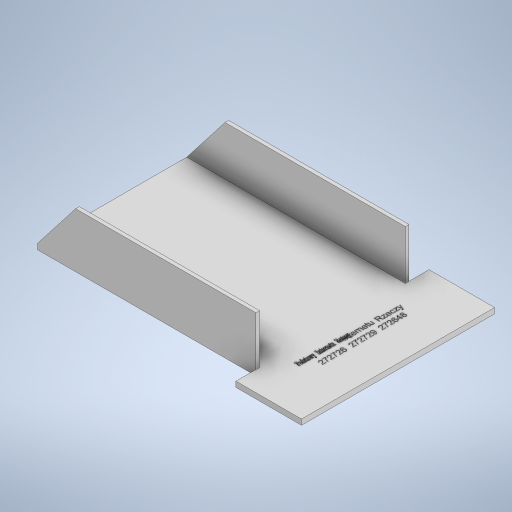
# Autodesk Inventor part: Część1
Saved by Autodesk Inventor 2024 (Build 280153020, 153B)
## iProperties
Created: 2025-01-23
Part Number: Część1
Material: Ogólny
Document SubType Name: Modeling
Designer: jakub
Density: 1 g/cm^3
Appearance: Domyślna
Author: jakub
Autodesk Inventor part; units mm, degrees
(part 1 of 2)
ref_plane "YZ Plane" through (0, 0, 0) normal (1, 0, 0) x (0, 1, 0)
ref_plane "XZ Plane" through (0, 0, 0) normal (0, 1, 0) x (-1, 0, 0)
ref_plane "XY Plane" through (0, 0, 0) normal (0, 0, 1) x (1, 0, 0)
sketch "Szkic1" plane through (0, 0, 0) normal (0, 1, 0) x (-1, 0, 0)
  line L0 (-24, 40) -> (60, 40)
  line L1 (60, -40) -> (-24, -40)
  line L2 (-60, -40) -> (-60, 40)
  line L3 (-60, 40) -> (60, -40) construction
  line L4 (60, 40) -> (-60, -40) construction
  line L5 (-24, -40) -> (-24, -53)
  line L6 (-24, -53) -> (-60, -53)
  line L7 (-60, -53) -> (-60, -40)
  line L8 (-24, 40) -> (-24, 53)
  line L9 (-24, 53) -> (-60, 53)
  line L10 (-60, 53) -> (-60, 40)
  line L11 (60, -40) -> (96, -40)
  line L12 (96, -40) -> (96, 40)
  line L13 (96, 40) -> (60, 40)
  point P0 (0, 0)
  dimension "d0" = 120
  dimension "d1" = 80
  dimension "d6" = 106
  dimension "d7" = 84
  dimension "d8" = 84
  dimension "d9" = 13
  dimension "d10" = 13
  dimension "d11" = 40
  dimension "d12" = 53
  dimension "d16" = 36
  dimension "d17" = 80
  dimension "d18" = 156
  constraints: 28 end point, 4 parallel, 2 horizontal, 2 midpoint, 1 perpendicular
  measures "d0" distance of L1.start L2.start
  measures "d1" distance of L0.end L1.start
  measures "d6" distance between parallel lines of L6 L9
  measures "d7" distance of L0.start L0.end
  measures "d8" distance of L1.start L1.end
  measures "d9" distance of L0.start L8.end
  measures "d10" distance of L1.end L5.end
  measures "d11" distance from line of point (0, 0) L1
  measures "d12" distance from line of point (0, 0) L9
  measures "d16" distance of L13.end L12.end
  measures "d17" distance of L11.end L12.end
  measures "d18" distance between parallel lines of L2 L12
extrude "Wyciągnięcie proste1" add sketch "Szkic1" along normal blind 3
sketch "Szkic2" plane through (0, 0, 0) normal (0, -1, 0) x (1, 0, 0)
  line L0 (24, -40) -> (-96, -40)
  line L1 (-96, -40) -> (-96, -42)
  line L2 (-96, -42) -> (24, -42)
  line L3 (24, -42) -> (24, -40)
  line L4 (24, 40) -> (-96, 40)
  line L5 (-96, 40) -> (-96, 42)
  line L6 (-96, 42) -> (24, 42)
  line L7 (24, 42) -> (24, 40)
  point P0 (0, 0)
  dimension "d19" = 2
  dimension "d20" = 120
  dimension "d21" = 2
  constraints: 16 end point, 4 parallel, 2 horizontal, 2 perpendicular, 1 point on line
  measures "d19" distance of L1.end L0.end
  measures "d20" distance of L5.end L6.end
  measures "d21" distance of L4.end L5.end
extrude "Wyciągnięcie proste2" add sketch "Szkic2" against normal blind 30
sketch "Szkic4" plane through (0, 3, 0) normal (0, 1, 0) x (1, 0, 0)
  line L0 (34.7111, -3.5872) -> (31.6611, -3.5872)
  line L1 (31.6611, -3.5872) -> (31.6611, -3.1828)
  line L2 (31.6611, -3.1828) -> (34.7111, -3.1828)
  line L3 (34.7111, -3.1828) -> (34.7111, -3.5872)
  line L4 (34.7111, -2.5202) -> (32.5003, -2.5202)
  line L5 (32.5003, -2.5202) -> (32.5003, -2.1831)
  line L6 (32.5003, -2.1831) -> (32.8141, -2.1831)
  spline S0 degree 2 poles (32.8141, -2.1831) (32.4515, -1.939) (32.4515, -1.4811) knots 0 0 0 1 1 1
  spline S1 degree 2 poles (32.4515, -1.4811) (32.4515, -1.2811) (32.5956, -0.9464) (32.8281, -0.779) (32.9885, -0.7465) knots 0 0 0 1 2 3 3 3
  spline S2 degree 2 poles (32.9885, -0.7465) (33.0931, -0.7255) (33.3534, -0.7255) knots 0 0 0 1 1 1
  line L7 (33.3534, -0.7255) -> (34.7111, -0.7255)
  line L8 (34.7111, -0.7255) -> (34.7111, -1.0998)
  line L9 (34.7111, -1.0998) -> (33.3674, -1.0998)
  spline S3 degree 2 poles (33.3674, -1.0998) (33.1396, -1.0998) (32.9117, -1.1882) (32.7769, -1.409) (32.7769, -1.5601) knots 0 0 0 1 2 3 3 3
  spline S4 degree 2 poles (32.7769, -1.5601) (32.7769, -1.7996) (33.0814, -2.1459) (33.5045, -2.1459) knots 0 0 0 1 2 2 2
  line L10 (33.5045, -2.1459) -> (34.7111, -2.1459)
  line L11 (34.7111, -2.1459) -> (34.7111, -2.5202)
  line L12 (34.3763, 0.6646) -> (34.7087, 0.7181)
  spline S5 degree 2 poles (34.7087, 0.7181) (34.7413, 0.56) (34.7413, 0.4345) knots 0 0 0 1 1 1
  spline S6 degree 2 poles (34.7413, 0.4345) (34.7413, 0.2322) (34.6111, 0.0067) (34.4019, -0.0839) (34.0648, -0.0839) knots 0 0 0 1 2 3 3 3
  line L13 (34.0648, -0.0839) -> (32.7909, -0.0839)
  line L14 (32.7909, -0.0839) -> (32.7909, -0.3606)
  line L15 (32.7909, -0.3606) -> (32.5003, -0.3606)
  line L16 (32.5003, -0.3606) -> (32.5003, -0.0839)
  line L17 (32.5003, -0.0839) -> (31.954, -0.0839)
  line L18 (31.954, -0.0839) -> (31.7285, 0.2903)
  line L19 (31.7285, 0.2903) -> (32.5003, 0.2903)
  line L20 (32.5003, 0.2903) -> (32.5003, 0.6646)
  line L21 (32.5003, 0.6646) -> (32.7909, 0.6646)
  line L22 (32.7909, 0.6646) -> (32.7909, 0.2903)
  line L23 (32.7909, 0.2903) -> (34.0857, 0.2903)
  spline S7 degree 2 poles (34.0857, 0.2903) (34.2461, 0.2903) (34.3391, 0.3299) (34.3926, 0.4182) (34.3926, 0.5019) knots 0 0 0 1 2 3 3 3
  spline S8 degree 2 poles (34.3926, 0.5019) (34.3926, 0.5623) (34.3763, 0.6646) knots 0 0 0 1 1 1
  line L24 (33.9974, 2.543) -> (34.0462, 2.9312)
  spline S9 degree 2 poles (34.0462, 2.9312) (34.3856, 2.8382) (34.7599, 2.3431) (34.7599, 1.9595) knots 0 0 0 1 2 2 2
  spline S10 degree 2 poles (34.7599, 1.9595) (34.7599, 1.4736) (34.1624, 0.9064) (33.6254, 0.9064) knots 0 0 0 1 2 2 2
  spline S11 degree 2 poles (33.6254, 0.9064) (33.0675, 0.9064) (32.4515, 1.4806) (32.4515, 1.9386) knots 0 0 0 1 2 2 2
  spline S12 degree 2 poles (32.4515, 1.9386) (32.4515, 2.3802) (33.0559, 2.9428) (33.6022, 2.9428) knots 0 0 0 1 2 2 2
  spline S13 degree 2 poles (33.6022, 2.9428) (33.6347, 2.9428) (33.7021, 2.9405) knots 0 0 0 1 1 1
  line L25 (33.7021, 2.9405) -> (33.7021, 1.2923)
  spline S14 degree 2 poles (33.7021, 1.2923) (34.0671, 1.3132) (34.453, 1.6828) (34.453, 1.9595) knots 0 0 0 1 2 2 2
  spline S15 degree 2 poles (34.453, 1.9595) (34.453, 2.1664) (34.2345, 2.457) (33.9974, 2.543) knots 0 0 0 1 2 2 2
  line L26 (33.3953, 1.3132) -> (33.3953, 2.5476)
  spline S16 degree 2 poles (33.3953, 2.5476) (33.1163, 2.5221) (32.9745, 2.4058) knots 0 0 0 1 1 1
  spline S17 degree 2 poles (32.9745, 2.4058) (32.7583, 2.2268) (32.7583, 1.9409) knots 0 0 0 1 1 1
  spline S18 degree 2 poles (32.7583, 1.9409) (32.7583, 1.6828) (33.1047, 1.3318) (33.3953, 1.3132) knots 0 0 0 1 2 2 2
  line L27 (34.7111, 3.3961) -> (32.5003, 3.3961)
  line L28 (32.5003, 3.3961) -> (32.5003, 3.7332)
  line L29 (32.5003, 3.7332) -> (32.835, 3.7332)
  spline S19 degree 2 poles (32.835, 3.7332) (32.6002, 3.8611) (32.4515, 4.0796) (32.4515, 4.2121) knots 0 0 0 1 2 2 2
  spline S20 degree 2 poles (32.4515, 4.2121) (32.4515, 4.4004) (32.57, 4.5957) knots 0 0 0 1 1 1
  line L30 (32.57, 4.5957) -> (32.9187, 4.4655)
  spline S21 degree 2 poles (32.9187, 4.4655) (32.8374, 4.3283) (32.8374, 4.1912) knots 0 0 0 1 1 1
  spline S22 degree 2 poles (32.8374, 4.1912) (32.8374, 4.068) (32.9861, 3.875) (33.1163, 3.8332) knots 0 0 0 1 2 2 2
  spline S23 degree 2 poles (33.1163, 3.8332) (33.3162, 3.7704) (33.5534, 3.7704) knots 0 0 0 1 1 1
  line L31 (33.5534, 3.7704) -> (34.7111, 3.7704)
  line L32 (34.7111, 3.7704) -> (34.7111, 3.3961)
  line L33 (34.7111, 4.8189) -> (32.5003, 4.8189)
  line L34 (32.5003, 4.8189) -> (32.5003, 5.1559)
  line L35 (32.5003, 5.1559) -> (32.8141, 5.1559)
  spline S24 degree 2 poles (32.8141, 5.1559) (32.4515, 5.4) (32.4515, 5.858) knots 0 0 0 1 1 1
  spline S25 degree 2 poles (32.4515, 5.858) (32.4515, 6.0579) (32.5956, 6.3927) (32.8281, 6.56) (32.9885, 6.5926) knots 0 0 0 1 2 3 3 3
  spline S26 degree 2 poles (32.9885, 6.5926) (33.0931, 6.6135) (33.3534, 6.6135) knots 0 0 0 1 1 1
  line L36 (33.3534, 6.6135) -> (34.7111, 6.6135)
  line L37 (34.7111, 6.6135) -> (34.7111, 6.2392)
  line L38 (34.7111, 6.2392) -> (33.3674, 6.2392)
  spline S27 degree 2 poles (33.3674, 6.2392) (33.1396, 6.2392) (32.9117, 6.1509) (32.7769, 5.9301) (32.7769, 5.7789) knots 0 0 0 1 2 3 3 3
  spline S28 degree 2 poles (32.7769, 5.7789) (32.7769, 5.5395) (33.0814, 5.1931) (33.5045, 5.1931) knots 0 0 0 1 2 2 2
  line L39 (33.5045, 5.1931) -> (34.7111, 5.1931)
  line L40 (34.7111, 5.1931) -> (34.7111, 4.8189)
  line L41 (33.9974, 8.6988) -> (34.0462, 9.087)
  spline S29 degree 2 poles (34.0462, 9.087) (34.3856, 8.994) (34.7599, 8.4988) (34.7599, 8.1153) knots 0 0 0 1 2 2 2
  spline S30 degree 2 poles (34.7599, 8.1153) (34.7599, 7.6294) (34.1624, 7.0622) (33.6254, 7.0622) knots 0 0 0 1 2 2 2
  spline S31 degree 2 poles (33.6254, 7.0622) (33.0675, 7.0622) (32.4515, 7.6364) (32.4515, 8.0943) knots 0 0 0 1 2 2 2
  spline S32 degree 2 poles (32.4515, 8.0943) (32.4515, 8.536) (33.0559, 9.0986) (33.6022, 9.0986) knots 0 0 0 1 2 2 2
  spline S33 degree 2 poles (33.6022, 9.0986) (33.6347, 9.0986) (33.7021, 9.0963) knots 0 0 0 1 1 1
  line L42 (33.7021, 9.0963) -> (33.7021, 7.4481)
  spline S34 degree 2 poles (33.7021, 7.4481) (34.0671, 7.469) (34.453, 7.8386) (34.453, 8.1153) knots 0 0 0 1 2 2 2
  spline S35 degree 2 poles (34.453, 8.1153) (34.453, 8.3222) (34.2345, 8.6128) (33.9974, 8.6988) knots 0 0 0 1 2 2 2
  line L43 (33.3953, 7.469) -> (33.3953, 8.7034)
  spline S36 degree 2 poles (33.3953, 8.7034) (33.1163, 8.6778) (32.9745, 8.5616) knots 0 0 0 1 1 1
  spline S37 degree 2 poles (32.9745, 8.5616) (32.7583, 8.3826) (32.7583, 8.0967) knots 0 0 0 1 1 1
  spline S38 degree 2 poles (32.7583, 8.0967) (32.7583, 7.8386) (33.1047, 7.4876) (33.3953, 7.469) knots 0 0 0 1 2 2 2
  line L44 (34.3763, 10.3725) -> (34.7087, 10.426)
  spline S39 degree 2 poles (34.7087, 10.426) (34.7413, 10.2679) (34.7413, 10.1424) knots 0 0 0 1 1 1
  spline S40 degree 2 poles (34.7413, 10.1424) (34.7413, 9.9402) (34.6111, 9.7147) (34.4019, 9.624) (34.0648, 9.624) knots 0 0 0 1 2 3 3 3
  line L45 (34.0648, 9.624) -> (32.7909, 9.624)
  line L46 (32.7909, 9.624) -> (32.7909, 9.3474)
  line L47 (32.7909, 9.3474) -> (32.5003, 9.3474)
  line L48 (32.5003, 9.3474) -> (32.5003, 9.624)
  line L49 (32.5003, 9.624) -> (31.954, 9.624)
  line L50 (31.954, 9.624) -> (31.7285, 9.9983)
  line L51 (31.7285, 9.9983) -> (32.5003, 9.9983)
  line L52 (32.5003, 9.9983) -> (32.5003, 10.3725)
  line L53 (32.5003, 10.3725) -> (32.7909, 10.3725)
  line L54 (32.7909, 10.3725) -> (32.7909, 9.9983)
  line L55 (32.7909, 9.9983) -> (34.0857, 9.9983)
  spline S41 degree 2 poles (34.0857, 9.9983) (34.2461, 9.9983) (34.3391, 10.0378) (34.3926, 10.1261) (34.3926, 10.2098) knots 0 0 0 1 2 3 3 3
  spline S42 degree 2 poles (34.3926, 10.2098) (34.3926, 10.2703) (34.3763, 10.3725) knots 0 0 0 1 1 1
  line L56 (34.7111, 12.1858) -> (34.3856, 12.1858)
  spline S43 degree 2 poles (34.3856, 12.1858) (34.7599, 11.9278) (34.7599, 11.4861) knots 0 0 0 1 1 1
  spline S44 degree 2 poles (34.7599, 11.4861) (34.7599, 11.2908) (34.6111, 10.9514) (34.3833, 10.7863) (34.2182, 10.7538) knots 0 0 0 1 2 3 3 3
  spline S45 degree 2 poles (34.2182, 10.7538) (34.109, 10.7306) (33.8695, 10.7306) knots 0 0 0 1 1 1
  line L57 (33.8695, 10.7306) -> (32.5003, 10.7306)
  line L58 (32.5003, 10.7306) -> (32.5003, 11.1048)
  line L59 (32.5003, 11.1048) -> (33.7254, 11.1048)
  spline S46 degree 2 poles (33.7254, 11.1048) (34.0183, 11.1048) (34.1206, 11.1281) knots 0 0 0 1 1 1
  spline S47 degree 2 poles (34.1206, 11.1281) (34.2694, 11.1629) (34.4367, 11.3908) (34.4367, 11.5605) knots 0 0 0 1 2 2 2
  spline S48 degree 2 poles (34.4367, 11.5605) (34.4367, 11.7278) (34.2647, 12.0231) (33.9672, 12.1463) (33.6835, 12.1463) knots 0 0 0 1 2 3 3 3
  line L60 (33.6835, 12.1463) -> (32.5003, 12.1463)
  line L61 (32.5003, 12.1463) -> (32.5003, 12.5206)
  line L62 (32.5003, 12.5206) -> (34.7111, 12.5206)
  line L63 (34.7111, 12.5206) -> (34.7111, 12.1858)
  line L64 (33.4322, -27.6981) -> (34.2484, -27.6981)
  line L65 (34.2484, -27.6981) -> (34.2484, -28.4374)
  line L66 (34.2484, -28.4374) -> (33.4322, -28.4374)
  line L67 (33.4322, -28.4374) -> (33.4322, -28.2904)
  line L68 (33.4322, -28.2904) -> (31.9784, -28.2904)
  line L69 (31.9784, -28.2904) -> (31.9784, -28.4374)
  line L70 (31.9784, -28.4374) -> (31.1984, -28.4374)
  line L71 (31.1984, -28.4374) -> (31.1984, -27.8269)
  spline S49 degree 2 poles (31.1984, -27.8269) (31.1984, -27.4335) (31.5737, -27.1713) (32.1321, -27.1713) knots 0 0 0 1 2 2 2
  spline S50 degree 2 poles (32.1321, -27.1713) (32.6205, -27.1713) (32.9348, -27.4064) (32.9348, -27.7681) knots 0 0 0 1 2 2 2
  line L72 (32.9348, -27.7681) -> (32.9348, -27.8631)
  line L73 (32.9348, -27.8631) -> (33.4322, -27.8631)
  line L74 (33.4322, -27.8631) -> (33.4322, -27.6981)
  line L75 (31.9784, -27.8631) -> (32.6002, -27.8631)
  line L76 (32.6002, -27.8631) -> (32.6002, -27.8314)
  line L77 (32.6002, -27.8314) -> (32.6002, -27.7727)
  spline S51 degree 2 poles (32.6002, -27.7727) (32.6002, -27.5827) (32.304, -27.5827) knots 0 0 0 1 1 1
  spline S52 degree 2 poles (32.304, -27.5827) (31.9784, -27.5827) (31.9784, -27.8021) knots 0 0 0 1 1 1
  line L78 (31.9784, -27.8021) -> (31.9784, -27.8631)
  line L79 (33.5023, -27.0266) -> (32.7675, -27.0266)
  spline S53 degree 2 poles (32.7675, -27.0266) (32.2723, -27.0266) (31.9467, -26.8457) (31.9467, -26.5676) knots 0 0 0 1 2 2 2
  spline S54 degree 2 poles (31.9467, -26.5676) (31.9467, -26.2918) (32.2814, -26.1086) (32.7901, -26.1086) knots 0 0 0 1 2 2 2
  line L80 (32.7901, -26.1086) -> (33.4729, -26.1086)
  line L81 (33.4729, -26.1086) -> (33.6515, -26.1109)
  spline S55 degree 2 poles (33.6515, -26.1109) (34.2755, -26.1109) (34.2755, -26.5744) knots 0 0 0 1 1 1
  spline S56 degree 2 poles (34.2755, -26.5744) (34.2755, -27.0266) (33.5023, -27.0266) knots 0 0 0 1 1 1
  line L82 (33.2129, -26.4274) -> (32.937, -26.4274)
  line L83 (32.937, -26.4274) -> (32.8353, -26.4297)
  line L84 (32.8353, -26.4297) -> (32.7449, -26.4297)
  spline S57 degree 2 poles (32.7449, -26.4297) (32.5572, -26.4297) (32.5572, -26.5653) knots 0 0 0 1 1 1
  spline S58 degree 2 poles (32.5572, -26.5653) (32.5572, -26.7078) (32.9551, -26.7078) knots 0 0 0 1 1 1
  line L85 (32.9551, -26.7078) -> (33.2445, -26.7078)
  spline S59 degree 2 poles (33.2445, -26.7078) (33.6108, -26.7078) (33.6108, -26.5698) knots 0 0 0 1 1 1
  spline S60 degree 2 poles (33.6108, -26.5698) (33.6108, -26.4274) (33.2129, -26.4274) knots 0 0 0 1 1 1
  line L86 (31.1984, -24.9849) -> (33.6063, -24.9849)
  line L87 (33.6063, -24.9849) -> (33.6063, -24.8674)
  line L88 (33.6063, -24.8674) -> (34.2484, -24.8674)
  line L89 (34.2484, -24.8674) -> (34.2484, -25.2495)
  line L90 (34.2484, -25.2495) -> (34.0381, -25.2495)
  spline S61 degree 2 poles (34.0381, -25.2495) (34.0698, -25.2969) (34.1263, -25.3309) knots 0 0 0 1 1 1
  spline S62 degree 2 poles (34.1263, -25.3309) (34.2778, -25.4213) (34.2778, -25.5773) knots 0 0 0 1 1 1
  spline S63 degree 2 poles (34.2778, -25.5773) (34.2778, -25.9051) (33.4819, -25.9051) knots 0 0 0 1 1 1
  line L91 (33.4819, -25.9051) -> (32.8353, -25.9051)
  spline S64 degree 2 poles (32.8353, -25.9051) (31.9467, -25.9051) (31.9467, -25.5818) knots 0 0 0 1 1 1
  spline S65 degree 2 poles (31.9467, -25.5818) (31.9467, -25.4009) (32.1683, -25.3037) knots 0 0 0 1 1 1
  line L92 (32.1683, -25.3037) -> (31.7094, -25.3037)
  line L93 (31.7094, -25.3037) -> (31.7094, -25.4349)
  line L94 (31.7094, -25.4349) -> (31.1984, -25.4349)
  line L95 (31.1984, -25.4349) -> (31.1984, -24.9849)
  spline S66 degree 2 poles (32.5572, -25.4371) (32.5482, -25.5683) (32.8466, -25.5683) knots 0 0 0 1 1 1
  line L96 (32.8466, -25.5683) -> (33.1157, -25.5705)
  line L97 (33.1157, -25.5705) -> (33.3644, -25.5705)
  spline S67 degree 2 poles (33.3644, -25.5705) (33.6741, -25.5705) (33.6673, -25.4371) knots 0 0 0 1 1 1
  spline S68 degree 2 poles (33.6673, -25.4371) (33.6605, -25.315) (33.2084, -25.315) knots 0 0 0 1 1 1
  spline S69 degree 2 poles (33.2084, -25.315) (32.5662, -25.315) (32.5572, -25.4371) knots 0 0 0 1 1 1
  line L98 (31.9784, -23.9223) -> (32.8556, -23.9223)
  line L99 (32.8556, -23.9223) -> (32.8556, -24.1823)
  line L100 (32.8556, -24.1823) -> (32.7946, -24.1823)
  spline S70 degree 2 poles (32.7946, -24.1823) (32.5595, -24.1823) (32.5595, -24.3496) knots 0 0 0 1 1 1
  spline S71 degree 2 poles (32.5595, -24.3496) (32.5595, -24.4807) (32.6906, -24.4807) knots 0 0 0 1 1 1
  spline S72 degree 2 poles (32.6906, -24.4807) (32.8014, -24.4807) (32.8669, -24.3654) knots 0 0 0 1 1 1
  line L101 (32.8669, -24.3654) -> (32.9642, -24.1959)
  spline S73 degree 2 poles (32.9642, -24.1959) (33.1563, -23.868) (33.5656, -23.868) knots 0 0 0 1 1 1
  spline S74 degree 2 poles (33.5656, -23.868) (34.2778, -23.868) (34.2778, -24.1868) knots 0 0 0 1 1 1
  spline S75 degree 2 poles (34.2778, -24.1868) (34.2778, -24.3993) (34.0381, -24.483) knots 0 0 0 1 1 1
  line L102 (34.0381, -24.483) -> (34.2484, -24.483)
  line L103 (34.2484, -24.483) -> (34.2484, -24.743)
  line L104 (34.2484, -24.743) -> (33.3191, -24.743)
  line L105 (33.3191, -24.743) -> (33.3191, -24.483)
  line L106 (33.3191, -24.483) -> (33.3644, -24.483)
  spline S76 degree 2 poles (33.3644, -24.483) (33.6673, -24.483) (33.6673, -24.3315) knots 0 0 0 1 1 1
  spline S77 degree 2 poles (33.6673, -24.3315) (33.6673, -24.1959) (33.5113, -24.1959) knots 0 0 0 1 1 1
  spline S78 degree 2 poles (33.5113, -24.1959) (33.3395, -24.1959) (33.2445, -24.3519) knots 0 0 0 1 1 1
  line L107 (33.2445, -24.3519) -> (33.179, -24.4627)
  spline S79 degree 2 poles (33.179, -24.4627) (32.989, -24.7769) (32.5662, -24.7769) knots 0 0 0 1 1 1
  spline S80 degree 2 poles (32.5662, -24.7769) (31.949, -24.7769) (31.949, -24.4717) knots 0 0 0 1 1 1
  spline S81 degree 2 poles (31.949, -24.4717) (31.949, -24.2773) (32.1977, -24.1823) knots 0 0 0 1 1 1
  line L108 (32.1977, -24.1823) -> (31.9784, -24.1823)
  line L109 (31.9784, -24.1823) -> (31.9784, -23.9223)
  line L110 (31.9784, -23.1332) -> (32.5889, -23.1332)
  line L111 (32.5889, -23.1332) -> (32.5889, -23.3435)
  line L112 (32.5889, -23.3435) -> (33.3644, -23.3435)
  line L113 (33.3644, -23.3435) -> (33.4774, -23.3412)
  spline S82 degree 2 poles (33.4774, -23.3412) (33.6696, -23.3412) (33.6696, -23.2124) knots 0 0 0 1 1 1
  spline S83 degree 2 poles (33.6696, -23.2124) (33.6696, -23.1581) (33.6108, -23.0744) knots 0 0 0 1 1 1
  line L114 (33.6108, -23.0744) -> (34.2212, -23.0744)
  spline S84 degree 2 poles (34.2212, -23.0744) (34.28, -23.2327) (34.28, -23.3164) knots 0 0 0 1 1 1
  spline S85 degree 2 poles (34.28, -23.3164) (34.28, -23.6691) (33.7487, -23.6691) knots 0 0 0 1 1 1
  line L115 (33.7487, -23.6691) -> (33.604, -23.6645)
  line L116 (33.604, -23.6645) -> (33.4548, -23.6623)
  line L117 (33.4548, -23.6623) -> (32.5889, -23.6623)
  line L118 (32.5889, -23.6623) -> (32.5889, -23.7821)
  line L119 (32.5889, -23.7821) -> (31.9784, -23.7821)
  spline S86 degree 2 poles (31.9784, -23.7821) (31.8201, -23.4995) (31.4132, -23.4678) knots 0 0 0 1 1 1
  line L120 (31.4132, -23.4678) -> (31.3159, -23.4588)
  spline S87 degree 2 poles (31.3159, -23.4588) (31.3092, -23.4588) (31.2775, -23.4543) knots 0 0 0 1 1 1
  line L121 (31.2775, -23.4543) -> (31.2775, -23.3435)
  line L122 (31.2775, -23.3435) -> (31.9784, -23.3435)
  line L123 (31.9784, -23.3435) -> (31.9784, -23.1332)
  line L124 (33.5904, -21.9146) -> (34.2212, -21.9146)
  spline S88 degree 2 poles (34.2212, -21.9146) (34.2778, -22.0073) (34.2778, -22.1) knots 0 0 0 1 1 1
  spline S89 degree 2 poles (34.2778, -22.1) (34.2778, -22.2967) (34.063, -22.3803) knots 0 0 0 1 1 1
  spline S90 degree 2 poles (34.063, -22.3803) (34.2778, -22.4572) (34.2778, -22.6336) knots 0 0 0 1 1 1
  spline S91 degree 2 poles (34.2778, -22.6336) (34.2778, -22.9501) (33.5204, -22.9501) knots 0 0 0 1 1 1
  spline S92 degree 2 poles (33.5204, -22.9501) (33.1224, -22.9501) (32.919, -22.5838) knots 0 0 0 1 1 1
  spline S93 degree 2 poles (32.919, -22.5838) (32.8195, -22.3984) (32.7019, -22.3984) knots 0 0 0 1 1 1
  spline S94 degree 2 poles (32.7019, -22.3984) (32.5572, -22.3984) (32.5572, -22.5115) knots 0 0 0 1 1 1
  spline S95 degree 2 poles (32.5572, -22.5115) (32.5572, -22.629) (32.7313, -22.629) knots 0 0 0 1 1 1
  spline S96 degree 2 poles (32.7313, -22.629) (32.7675, -22.629) (32.8376, -22.6177) knots 0 0 0 1 1 1
  line L125 (32.8376, -22.6177) -> (32.8376, -22.923)
  spline S97 degree 2 poles (32.8376, -22.923) (32.6906, -22.9569) (32.4939, -22.9569) knots 0 0 0 1 1 1
  spline S98 degree 2 poles (32.4939, -22.9569) (31.9467, -22.9569) (31.9467, -22.4934) knots 0 0 0 1 1 1
  spline S99 degree 2 poles (31.9467, -22.4934) (31.9467, -22.0615) (32.512, -22.0615) knots 0 0 0 1 1 1
  line L126 (32.512, -22.0615) -> (32.6929, -22.0615)
  line L127 (32.6929, -22.0615) -> (33.3395, -22.0615)
  spline S100 degree 2 poles (33.3395, -22.0615) (33.6131, -22.0615) (33.6131, -21.9688) knots 0 0 0 1 1 1
  spline S101 degree 2 poles (33.6131, -21.9688) (33.6131, -21.9508) (33.5904, -21.9146) knots 0 0 0 1 1 1
  spline S102 degree 2 poles (33.1405, -22.3803) (33.2762, -22.6539) (33.4571, -22.6539) knots 0 0 0 1 1 1
  spline S103 degree 2 poles (33.4571, -22.6539) (33.6131, -22.6539) (33.6131, -22.5205) knots 0 0 0 1 1 1
  spline S104 degree 2 poles (33.6131, -22.5205) (33.6131, -22.3803) (33.3395, -22.3803) knots 0 0 0 1 1 1
  line L128 (33.3395, -22.3803) -> (33.1405, -22.3803)
  line L129 (31.9784, -20.0787) -> (32.5889, -20.0787)
  line L130 (32.5889, -20.0787) -> (32.5889, -20.1895)
  line L131 (32.5889, -20.1895) -> (34.2484, -20.4495)
  line L132 (34.2484, -20.4495) -> (34.2484, -20.7886)
  line L133 (34.2484, -20.7886) -> (33.0139, -20.9288)
  line L134 (33.0139, -20.9288) -> (34.2484, -21.1006)
  line L135 (34.2484, -21.1006) -> (34.2484, -21.4601)
  line L136 (34.2484, -21.4601) -> (32.5889, -21.7314)
  line L137 (32.5889, -21.7314) -> (32.5889, -21.8468)
  line L138 (32.5889, -21.8468) -> (31.9784, -21.8468)
  line L139 (31.9784, -21.8468) -> (31.9784, -21.3064)
  line L140 (31.9784, -21.3064) -> (32.5889, -21.3064)
  line L141 (32.5889, -21.3064) -> (32.5889, -21.4194)
  line L142 (32.5889, -21.4194) -> (33.7261, -21.2589)
  line L143 (33.7261, -21.2589) -> (32.5889, -21.1006)
  line L144 (32.5889, -21.1006) -> (32.5889, -21.2114)
  line L145 (32.5889, -21.2114) -> (31.9784, -21.2114)
  line L146 (31.9784, -21.2114) -> (31.9784, -20.6394)
  line L147 (31.9784, -20.6394) -> (32.5889, -20.6394)
  line L148 (32.5889, -20.6394) -> (32.5889, -20.7479)
  line L149 (32.5889, -20.7479) -> (33.7261, -20.601)
  line L150 (33.7261, -20.601) -> (32.5889, -20.4495)
  line L151 (32.5889, -20.4495) -> (32.5889, -20.558)
  line L152 (32.5889, -20.558) -> (31.9784, -20.558)
  line L153 (31.9784, -20.558) -> (31.9784, -20.0787)
  line L154 (31.9784, -18.9075) -> (32.5889, -18.9075)
  line L155 (32.5889, -18.9075) -> (32.5889, -19.0161)
  line L156 (32.5889, -19.0161) -> (34.3411, -19.2648)
  spline S105 degree 2 poles (34.3411, -19.2648) (35.0668, -19.3688) (35.0668, -19.6876) knots 0 0 0 1 1 1
  spline S106 degree 2 poles (35.0668, -19.6876) (35.0668, -20.0131) (34.6147, -20.0131) knots 0 0 0 1 1 1
  spline S107 degree 2 poles (34.6147, -20.0131) (34.4632, -20.0131) (34.2959, -19.9883) knots 0 0 0 1 1 1
  line L157 (34.2959, -19.9883) -> (34.2959, -19.7757)
  spline S108 degree 2 poles (34.2959, -19.7757) (34.3592, -19.7848) (34.4044, -19.7848) knots 0 0 0 1 1 1
  spline S109 degree 2 poles (34.4044, -19.7848) (34.54, -19.7848) (34.54, -19.6921) knots 0 0 0 1 1 1
  spline S110 degree 2 poles (34.54, -19.6921) (34.54, -19.6062) (34.2959, -19.5609) knots 0 0 0 1 1 1
  line L158 (34.2959, -19.5609) -> (32.5889, -19.8956)
  line L159 (32.5889, -19.8956) -> (32.5889, -20.0109)
  line L160 (32.5889, -20.0109) -> (31.9784, -20.0109)
  line L161 (31.9784, -20.0109) -> (31.9784, -19.4705)
  line L162 (31.9784, -19.4705) -> (32.5889, -19.4705)
  line L163 (32.5889, -19.4705) -> (32.5889, -19.5836)
  line L164 (32.5889, -19.5836) -> (33.5769, -19.3869)
  line L165 (33.5769, -19.3869) -> (32.5889, -19.2648)
  line L166 (32.5889, -19.2648) -> (32.5889, -19.3869)
  line L167 (32.5889, -19.3869) -> (31.9784, -19.3869)
  line L168 (31.9784, -19.3869) -> (31.9784, -18.9075)
  line L169 (31.1984, -16.6715) -> (31.9784, -16.6715)
  line L170 (31.9784, -16.6715) -> (31.9784, -16.832)
  line L171 (31.9784, -16.832) -> (33.4322, -16.832)
  line L172 (33.4322, -16.832) -> (33.4322, -16.6715)
  line L173 (33.4322, -16.6715) -> (34.2484, -16.6715)
  line L174 (34.2484, -16.6715) -> (34.2484, -17.4108)
  line L175 (34.2484, -17.4108) -> (33.4322, -17.4108)
  line L176 (33.4322, -17.4108) -> (33.4322, -17.2593)
  line L177 (33.4322, -17.2593) -> (31.9784, -17.2593)
  line L178 (31.9784, -17.2593) -> (31.9784, -17.4108)
  line L179 (31.9784, -17.4108) -> (31.1984, -17.4108)
  line L180 (31.1984, -17.4108) -> (31.1984, -16.6715)
  line L181 (33.6063, -15.3534) -> (34.2484, -15.3534)
  line L182 (34.2484, -15.3534) -> (34.2484, -15.8937)
  line L183 (34.2484, -15.8937) -> (33.6063, -15.8937)
  line L184 (33.6063, -15.8937) -> (33.6063, -15.801)
  line L185 (33.6063, -15.801) -> (32.9574, -15.801)
  line L186 (32.9574, -15.801) -> (32.876, -15.801)
  line L187 (32.876, -15.801) -> (32.7765, -15.8033)
  spline S111 degree 2 poles (32.7765, -15.8033) (32.5572, -15.8033) (32.5572, -15.905) knots 0 0 0 1 1 1
  spline S112 degree 2 poles (32.5572, -15.905) (32.5572, -16.0814) (32.9732, -16.0814) knots 0 0 0 1 1 1
  line L188 (32.9732, -16.0814) -> (33.6063, -16.0814)
  line L189 (33.6063, -16.0814) -> (33.6063, -15.9683)
  line L190 (33.6063, -15.9683) -> (34.2484, -15.9683)
  line L191 (34.2484, -15.9683) -> (34.2484, -16.5087)
  line L192 (34.2484, -16.5087) -> (33.6063, -16.5087)
  line L193 (33.6063, -16.5087) -> (33.6063, -16.3889)
  line L194 (33.6063, -16.3889) -> (32.5889, -16.3889)
  line L195 (32.5889, -16.3889) -> (32.5889, -16.5087)
  line L196 (32.5889, -16.5087) -> (31.9784, -16.5087)
  line L197 (31.9784, -16.5087) -> (31.9784, -16.0814)
  line L198 (31.9784, -16.0814) -> (32.2565, -16.0814)
  spline S113 degree 2 poles (32.2565, -16.0814) (31.9467, -15.9615) (31.9467, -15.7558) knots 0 0 0 1 1 1
  spline S114 degree 2 poles (31.9467, -15.7558) (31.9467, -15.4822) (32.4193, -15.4822) knots 0 0 0 1 1 1
  line L199 (32.4193, -15.4822) -> (32.5889, -15.4822)
  line L200 (32.5889, -15.4822) -> (33.6063, -15.4822)
  line L201 (33.6063, -15.4822) -> (33.6063, -15.3534)
  line L202 (31.9784, -14.6412) -> (32.5889, -14.6412)
  line L203 (32.5889, -14.6412) -> (32.5889, -14.8514)
  line L204 (32.5889, -14.8514) -> (33.3644, -14.8514)
  line L205 (33.3644, -14.8514) -> (33.4774, -14.8492)
  spline S115 degree 2 poles (33.4774, -14.8492) (33.6696, -14.8492) (33.6696, -14.7203) knots 0 0 0 1 1 1
  spline S116 degree 2 poles (33.6696, -14.7203) (33.6696, -14.666) (33.6108, -14.5824) knots 0 0 0 1 1 1
  line L206 (33.6108, -14.5824) -> (34.2212, -14.5824)
  spline S117 degree 2 poles (34.2212, -14.5824) (34.28, -14.7406) (34.28, -14.8243) knots 0 0 0 1 1 1
  spline S118 degree 2 poles (34.28, -14.8243) (34.28, -15.177) (33.7487, -15.177) knots 0 0 0 1 1 1
  line L207 (33.7487, -15.177) -> (33.604, -15.1725)
  line L208 (33.604, -15.1725) -> (33.4548, -15.1702)
  line L209 (33.4548, -15.1702) -> (32.5889, -15.1702)
  line L210 (32.5889, -15.1702) -> (32.5889, -15.29)
  line L211 (32.5889, -15.29) -> (31.9784, -15.29)
  spline S119 degree 2 poles (31.9784, -15.29) (31.8201, -15.0074) (31.4132, -14.9758) knots 0 0 0 1 1 1
  line L212 (31.4132, -14.9758) -> (31.3159, -14.9667)
  spline S120 degree 2 poles (31.3159, -14.9667) (31.3092, -14.9667) (31.2775, -14.9622) knots 0 0 0 1 1 1
  line L213 (31.2775, -14.9622) -> (31.2775, -14.8514)
  line L214 (31.2775, -14.8514) -> (31.9784, -14.8514)
  line L215 (31.9784, -14.8514) -> (31.9784, -14.6412)
  spline S121 degree 2 poles (33.2739, -13.574) (33.4028, -13.5582) (33.5837, -13.5582) knots 0 0 0 1 1 1
  spline S122 degree 2 poles (33.5837, -13.5582) (34.2755, -13.5582) (34.2755, -13.9832) knots 0 0 0 1 1 1
  spline S123 degree 2 poles (34.2755, -13.9832) (34.2755, -14.2794) (33.8098, -14.4512) (33.0049, -14.4512) knots 0 0 0 1 2 2 2
  spline S124 degree 2 poles (33.0049, -14.4512) (32.3899, -14.4512) (31.9467, -14.2613) (31.9467, -13.9968) knots 0 0 0 1 2 2 2
  spline S125 degree 2 poles (31.9467, -13.9968) (31.9467, -13.7368) (32.4035, -13.5446) (33.0184, -13.5446) knots 0 0 0 1 2 2 2
  line L216 (33.0184, -13.5446) -> (33.1699, -13.5469)
  line L217 (33.1699, -13.5469) -> (33.1699, -14.1121)
  line L218 (33.1699, -14.1121) -> (33.396, -14.1121)
  line L219 (33.396, -14.1121) -> (33.5045, -14.1053)
  spline S126 degree 2 poles (33.5045, -14.1053) (33.6153, -14.0895) (33.6108, -13.9923) knots 0 0 0 1 1 1
  spline S127 degree 2 poles (33.6108, -13.9923) (33.6063, -13.8815) (33.396, -13.8815) knots 0 0 0 1 1 1
  line L220 (33.396, -13.8815) -> (33.3237, -13.8815)
  line L221 (33.3237, -13.8815) -> (33.2739, -13.8792)
  line L222 (33.2739, -13.8792) -> (33.2739, -13.574)
  line L223 (32.9167, -14.1189) -> (32.9167, -13.8792)
  line L224 (32.9167, -13.8792) -> (32.7539, -13.8792)
  spline S128 degree 2 poles (32.7539, -13.8792) (32.5572, -13.8792) (32.5572, -13.9991) knots 0 0 0 1 1 1
  spline S129 degree 2 poles (32.5572, -13.9991) (32.5572, -14.1234) (32.7946, -14.1234) knots 0 0 0 1 1 1
  spline S130 degree 2 poles (32.7946, -14.1234) (32.8421, -14.1234) (32.9167, -14.1189) knots 0 0 0 1 1 1
  line L225 (31.9784, -13.3705) -> (31.9784, -12.9342)
  line L226 (31.9784, -12.9342) -> (32.2542, -12.9342)
  spline S131 degree 2 poles (32.2542, -12.9342) (31.9467, -12.8618) (31.9467, -12.7126) knots 0 0 0 1 1 1
  spline S132 degree 2 poles (31.9467, -12.7126) (31.9467, -12.482) (32.4735, -12.482) knots 0 0 0 1 1 1
  spline S133 degree 2 poles (32.4735, -12.482) (32.8195, -12.482) (33.0591, -12.5068) knots 0 0 0 1 1 1
  line L227 (33.0591, -12.5068) -> (33.0591, -12.7646)
  spline S134 degree 2 poles (33.0591, -12.7646) (32.9303, -12.7488) (32.876, -12.7488) knots 0 0 0 1 1 1
  spline S135 degree 2 poles (32.876, -12.7488) (32.5572, -12.7488) (32.5572, -12.855) knots 0 0 0 1 1 1
  spline S136 degree 2 poles (32.5572, -12.855) (32.5572, -12.9342) (32.8466, -12.9342) knots 0 0 0 1 1 1
  line L228 (32.8466, -12.9342) -> (33.6063, -12.9342)
  line L229 (33.6063, -12.9342) -> (33.6063, -12.7985)
  line L230 (33.6063, -12.7985) -> (34.2484, -12.7985)
  line L231 (34.2484, -12.7985) -> (34.2484, -13.3705)
  line L232 (34.2484, -13.3705) -> (33.6063, -13.3705)
  line L233 (33.6063, -13.3705) -> (33.6063, -13.2529)
  line L234 (33.6063, -13.2529) -> (32.5889, -13.2529)
  line L235 (32.5889, -13.2529) -> (32.5889, -13.3705)
  line L236 (32.5889, -13.3705) -> (31.9784, -13.3705)
  line L237 (33.6063, -11.2158) -> (34.2484, -11.2158)
  line L238 (34.2484, -11.2158) -> (34.2484, -11.7562)
  line L239 (34.2484, -11.7562) -> (33.6063, -11.7562)
  line L240 (33.6063, -11.7562) -> (33.6063, -11.6635)
  line L241 (33.6063, -11.6635) -> (32.9574, -11.6635)
  line L242 (32.9574, -11.6635) -> (32.876, -11.6635)
  line L243 (32.876, -11.6635) -> (32.7765, -11.6658)
  spline S137 degree 2 poles (32.7765, -11.6658) (32.5572, -11.6658) (32.5572, -11.7675) knots 0 0 0 1 1 1
  spline S138 degree 2 poles (32.5572, -11.7675) (32.5572, -11.9439) (32.9732, -11.9439) knots 0 0 0 1 1 1
  line L244 (32.9732, -11.9439) -> (33.6063, -11.9439)
  line L245 (33.6063, -11.9439) -> (33.6063, -11.8308)
  line L246 (33.6063, -11.8308) -> (34.2484, -11.8308)
  line L247 (34.2484, -11.8308) -> (34.2484, -12.3712)
  line L248 (34.2484, -12.3712) -> (33.6063, -12.3712)
  line L249 (33.6063, -12.3712) -> (33.6063, -12.2513)
  line L250 (33.6063, -12.2513) -> (32.5889, -12.2513)
  line L251 (32.5889, -12.2513) -> (32.5889, -12.3712)
  line L252 (32.5889, -12.3712) -> (31.9784, -12.3712)
  line L253 (31.9784, -12.3712) -> (31.9784, -11.9439)
  line L254 (31.9784, -11.9439) -> (32.2565, -11.9439)
  spline S139 degree 2 poles (32.2565, -11.9439) (31.9467, -11.824) (31.9467, -11.6183) knots 0 0 0 1 1 1
  spline S140 degree 2 poles (31.9467, -11.6183) (31.9467, -11.3447) (32.4193, -11.3447) knots 0 0 0 1 1 1
  line L255 (32.4193, -11.3447) -> (32.5889, -11.3447)
  line L256 (32.5889, -11.3447) -> (33.6063, -11.3447)
  line L257 (33.6063, -11.3447) -> (33.6063, -11.2158)
  spline S141 degree 2 poles (33.2739, -10.2097) (33.4028, -10.1939) (33.5837, -10.1939) knots 0 0 0 1 1 1
  spline S142 degree 2 poles (33.5837, -10.1939) (34.2755, -10.1939) (34.2755, -10.619) knots 0 0 0 1 1 1
  spline S143 degree 2 poles (34.2755, -10.619) (34.2755, -10.9151) (33.8098, -11.087) (33.0049, -11.087) knots 0 0 0 1 2 2 2
  spline S144 degree 2 poles (33.0049, -11.087) (32.3899, -11.087) (31.9467, -10.8971) (31.9467, -10.6325) knots 0 0 0 1 2 2 2
  spline S145 degree 2 poles (31.9467, -10.6325) (31.9467, -10.3725) (32.4035, -10.1803) (33.0184, -10.1803) knots 0 0 0 1 2 2 2
  line L258 (33.0184, -10.1803) -> (33.1699, -10.1826)
  line L259 (33.1699, -10.1826) -> (33.1699, -10.7478)
  line L260 (33.1699, -10.7478) -> (33.396, -10.7478)
  line L261 (33.396, -10.7478) -> (33.5045, -10.741)
  spline S146 degree 2 poles (33.5045, -10.741) (33.6153, -10.7252) (33.6108, -10.628) knots 0 0 0 1 1 1
  spline S147 degree 2 poles (33.6108, -10.628) (33.6063, -10.5172) (33.396, -10.5172) knots 0 0 0 1 1 1
  line L262 (33.396, -10.5172) -> (33.3237, -10.5172)
  line L263 (33.3237, -10.5172) -> (33.2739, -10.515)
  line L264 (33.2739, -10.515) -> (33.2739, -10.2097)
  line L265 (32.9167, -10.7546) -> (32.9167, -10.515)
  line L266 (32.9167, -10.515) -> (32.7539, -10.515)
  spline S148 degree 2 poles (32.7539, -10.515) (32.5572, -10.515) (32.5572, -10.6348) knots 0 0 0 1 1 1
  spline S149 degree 2 poles (32.5572, -10.6348) (32.5572, -10.7591) (32.7946, -10.7591) knots 0 0 0 1 1 1
  spline S150 degree 2 poles (32.7946, -10.7591) (32.8421, -10.7591) (32.9167, -10.7546) knots 0 0 0 1 1 1
  line L267 (31.9784, -9.4026) -> (32.5889, -9.4026)
  line L268 (32.5889, -9.4026) -> (32.5889, -9.6128)
  line L269 (32.5889, -9.6128) -> (33.3644, -9.6128)
  line L270 (33.3644, -9.6128) -> (33.4774, -9.6106)
  spline S151 degree 2 poles (33.4774, -9.6106) (33.6696, -9.6106) (33.6696, -9.4817) knots 0 0 0 1 1 1
  spline S152 degree 2 poles (33.6696, -9.4817) (33.6696, -9.4274) (33.6108, -9.3438) knots 0 0 0 1 1 1
  line L271 (33.6108, -9.3438) -> (34.2212, -9.3438)
  spline S153 degree 2 poles (34.2212, -9.3438) (34.28, -9.5021) (34.28, -9.5857) knots 0 0 0 1 1 1
  spline S154 degree 2 poles (34.28, -9.5857) (34.28, -9.9384) (33.7487, -9.9384) knots 0 0 0 1 1 1
  line L272 (33.7487, -9.9384) -> (33.604, -9.9339)
  line L273 (33.604, -9.9339) -> (33.4548, -9.9316)
  line L274 (33.4548, -9.9316) -> (32.5889, -9.9316)
  line L275 (32.5889, -9.9316) -> (32.5889, -10.0515)
  line L276 (32.5889, -10.0515) -> (31.9784, -10.0515)
  spline S155 degree 2 poles (31.9784, -10.0515) (31.8201, -9.7688) (31.4132, -9.7372) knots 0 0 0 1 1 1
  line L277 (31.4132, -9.7372) -> (31.3159, -9.7281)
  spline S156 degree 2 poles (31.3159, -9.7281) (31.3092, -9.7281) (31.2775, -9.7236) knots 0 0 0 1 1 1
  line L278 (31.2775, -9.7236) -> (31.2775, -9.6128)
  line L279 (31.2775, -9.6128) -> (31.9784, -9.6128)
  line L280 (31.9784, -9.6128) -> (31.9784, -9.4026)
  line L281 (31.9784, -8.2382) -> (33.6063, -8.2382)
  line L282 (33.6063, -8.2382) -> (33.6063, -8.1093)
  line L283 (33.6063, -8.1093) -> (34.2484, -8.1093)
  line L284 (34.2484, -8.1093) -> (34.2484, -8.5366)
  line L285 (34.2484, -8.5366) -> (33.968, -8.5366)
  spline S157 degree 2 poles (33.968, -8.5366) (34.2755, -8.618) (34.2755, -8.8396) knots 0 0 0 1 1 1
  spline S158 degree 2 poles (34.2755, -8.8396) (34.2755, -9.1539) (33.6583, -9.1539) knots 0 0 0 1 1 1
  line L286 (33.6583, -9.1539) -> (32.5889, -9.1539)
  line L287 (32.5889, -9.1539) -> (32.5889, -9.276)
  line L288 (32.5889, -9.276) -> (31.9784, -9.276)
  line L289 (31.9784, -9.276) -> (31.9784, -8.8351)
  line L290 (31.9784, -8.8351) -> (33.301, -8.8351)
  spline S159 degree 2 poles (33.301, -8.8351) (33.6651, -8.8351) (33.6651, -8.7062) knots 0 0 0 1 1 1
  spline S160 degree 2 poles (33.6651, -8.7062) (33.6651, -8.557) (33.1948, -8.557) knots 0 0 0 1 1 1
  line L291 (33.1948, -8.557) -> (33.0772, -8.557)
  line L292 (33.0772, -8.557) -> (32.5889, -8.557)
  line L293 (32.5889, -8.557) -> (32.5889, -8.6881)
  line L294 (32.5889, -8.6881) -> (31.9784, -8.6881)
  line L295 (31.9784, -8.6881) -> (31.9784, -8.2382)
  spline S161 degree 2 poles (33.1111, -5.0864) (33.3689, -5.0616) (33.5498, -5.0616) knots 0 0 0 1 1 1
  spline S162 degree 2 poles (33.5498, -5.0616) (34.271, -5.0616) (34.271, -5.4052) knots 0 0 0 1 1 1
  spline S163 degree 2 poles (34.271, -5.4052) (34.271, -5.7353) (33.5204, -5.7353) knots 0 0 0 1 1 1
  line L296 (33.5204, -5.7353) -> (33.3191, -5.7331)
  line L297 (33.3191, -5.7331) -> (33.1157, -5.7308)
  spline S164 degree 2 poles (33.1157, -5.7308) (32.8398, -5.7308) (32.8398, -5.9931) knots 0 0 0 1 1 1
  spline S165 degree 2 poles (32.8398, -5.9931) (32.8398, -6.0021) (32.8421, -6.0338) knots 0 0 0 1 1 1
  line L298 (32.8421, -6.0338) -> (33.4322, -6.0338)
  line L299 (33.4322, -6.0338) -> (33.4322, -5.8733)
  line L300 (33.4322, -5.8733) -> (34.2484, -5.8733)
  line L301 (34.2484, -5.8733) -> (34.2484, -6.6126)
  line L302 (34.2484, -6.6126) -> (33.4322, -6.6126)
  line L303 (33.4322, -6.6126) -> (33.4322, -6.4611)
  line L304 (33.4322, -6.4611) -> (31.9784, -6.4611)
  line L305 (31.9784, -6.4611) -> (31.9784, -6.6126)
  line L306 (31.9784, -6.6126) -> (31.1984, -6.6126)
  line L307 (31.1984, -6.6126) -> (31.1984, -5.9207)
  spline S166 degree 2 poles (31.1984, -5.9207) (31.1984, -5.5432) (31.5217, -5.2877) (32.0033, -5.2877) knots 0 0 0 1 2 2 2
  spline S167 degree 2 poles (32.0033, -5.2877) (32.5866, -5.2877) (32.6702, -5.6426) knots 0 0 0 1 1 1
  spline S168 degree 2 poles (32.6702, -5.6426) (32.6748, -5.6607) (32.6816, -5.6946) knots 0 0 0 1 1 1
  spline S169 degree 2 poles (32.6816, -5.6946) (32.7336, -5.3917) (32.9574, -5.3758) knots 0 0 0 1 1 1
  line L308 (32.9574, -5.3758) -> (33.1677, -5.3645)
  line L309 (33.1677, -5.3645) -> (33.335, -5.3555)
  spline S170 degree 2 poles (33.335, -5.3555) (33.4616, -5.3487) (33.4616, -5.2832) knots 0 0 0 1 1 1
  spline S171 degree 2 poles (33.4616, -5.2832) (33.4616, -5.1927) (33.1609, -5.1927) knots 0 0 0 1 1 1
  line L310 (33.1609, -5.1927) -> (33.1111, -5.1927)
  line L311 (33.1111, -5.1927) -> (33.1111, -5.0864)
  line L312 (32.5414, -6.0338) -> (32.5414, -5.984)
  spline S172 degree 2 poles (32.5414, -5.984) (32.5414, -5.6992) (32.2768, -5.6992) knots 0 0 0 1 1 1
  spline S173 degree 2 poles (32.2768, -5.6992) (31.9761, -5.6992) (31.9761, -5.975) knots 0 0 0 1 1 1
  spline S174 degree 2 poles (31.9761, -5.975) (31.9761, -5.9931) (31.9784, -6.0338) knots 0 0 0 1 1 1
  line L313 (31.9784, -6.0338) -> (32.5414, -6.0338)
  line L314 (31.9784, -4.0622) -> (32.5889, -4.0622)
  line L315 (32.5889, -4.0622) -> (33.6063, -4.6614)
  line L316 (33.6063, -4.6614) -> (33.6063, -4.3223)
  line L317 (33.6063, -4.3223) -> (33.3191, -4.3223)
  line L318 (33.3191, -4.3223) -> (33.3191, -4.0622)
  line L319 (33.3191, -4.0622) -> (34.2484, -4.0622)
  line L320 (34.2484, -4.0622) -> (34.2484, -5.0073)
  line L321 (34.2484, -5.0073) -> (33.5746, -5.0073)
  line L322 (33.5746, -5.0073) -> (32.5889, -4.3856)
  line L323 (32.5889, -4.3856) -> (32.5889, -4.7134)
  line L324 (32.5889, -4.7134) -> (32.8556, -4.7134)
  line L325 (32.8556, -4.7134) -> (32.8556, -4.9734)
  line L326 (32.8556, -4.9734) -> (31.9784, -4.9734)
  line L327 (31.9784, -4.9734) -> (31.9784, -4.0622)
  spline S175 degree 2 poles (33.2739, -3.0222) (33.4028, -3.0064) (33.5837, -3.0064) knots 0 0 0 1 1 1
  spline S176 degree 2 poles (33.5837, -3.0064) (34.2755, -3.0064) (34.2755, -3.4314) knots 0 0 0 1 1 1
  spline S177 degree 2 poles (34.2755, -3.4314) (34.2755, -3.7276) (33.8098, -3.8995) (33.0049, -3.8995) knots 0 0 0 1 2 2 2
  spline S178 degree 2 poles (33.0049, -3.8995) (32.3899, -3.8995) (31.9467, -3.7095) (31.9467, -3.445) knots 0 0 0 1 2 2 2
  spline S179 degree 2 poles (31.9467, -3.445) (31.9467, -3.185) (32.4035, -2.9928) (33.0184, -2.9928) knots 0 0 0 1 2 2 2
  line L328 (33.0184, -2.9928) -> (33.1699, -2.9951)
  line L329 (33.1699, -2.9951) -> (33.1699, -3.5603)
  line L330 (33.1699, -3.5603) -> (33.396, -3.5603)
  line L331 (33.396, -3.5603) -> (33.5045, -3.5535)
  spline S180 degree 2 poles (33.5045, -3.5535) (33.6153, -3.5377) (33.6108, -3.4405) knots 0 0 0 1 1 1
  spline S181 degree 2 poles (33.6108, -3.4405) (33.6063, -3.3297) (33.396, -3.3297) knots 0 0 0 1 1 1
  line L332 (33.396, -3.3297) -> (33.3237, -3.3297)
  line L333 (33.3237, -3.3297) -> (33.2739, -3.3274)
  line L334 (33.2739, -3.3274) -> (33.2739, -3.0222)
  line L335 (32.9167, -3.5671) -> (32.9167, -3.3274)
  line L336 (32.9167, -3.3274) -> (32.7539, -3.3274)
  spline S182 degree 2 poles (32.7539, -3.3274) (32.5572, -3.3274) (32.5572, -3.4473) knots 0 0 0 1 1 1
  spline S183 degree 2 poles (32.5572, -3.4473) (32.5572, -3.5716) (32.7946, -3.5716) knots 0 0 0 1 1 1
  spline S184 degree 2 poles (32.7946, -3.5716) (32.8421, -3.5716) (32.9167, -3.5671) knots 0 0 0 1 1 1
  line L337 (33.1857, -1.937) -> (33.249, -1.9347)
  line L338 (33.249, -1.9347) -> (33.3553, -1.9347)
  line L339 (33.3553, -1.9347) -> (33.552, -1.9302)
  line L340 (33.552, -1.9302) -> (33.6696, -1.9324)
  spline S185 degree 2 poles (33.6696, -1.9324) (34.2755, -1.9324) (34.2755, -2.353) knots 0 0 0 1 1 1
  spline S186 degree 2 poles (34.2755, -2.353) (34.2755, -2.6107) (33.8572, -2.7984) (33.2762, -2.7984) knots 0 0 0 1 2 2 2
  line L341 (33.2762, -2.7984) -> (32.8647, -2.7984)
  spline S187 degree 2 poles (32.8647, -2.7984) (31.9467, -2.7984) (31.9467, -2.3598) knots 0 0 0 1 1 1
  spline S188 degree 2 poles (31.9467, -2.3598) (31.9467, -1.9347) (32.6182, -1.9347) knots 0 0 0 1 1 1
  spline S189 degree 2 poles (32.6182, -1.9347) (32.7675, -1.9347) (32.98, -1.9618) knots 0 0 0 1 1 1
  line L342 (32.98, -1.9618) -> (32.98, -2.2309)
  line L343 (32.98, -2.2309) -> (32.9031, -2.2309)
  line L344 (32.9031, -2.2309) -> (32.8217, -2.2309)
  line L345 (32.8217, -2.2309) -> (32.7652, -2.2309)
  line L346 (32.7652, -2.2309) -> (32.6431, -2.2422)
  spline S190 degree 2 poles (32.6431, -2.2422) (32.5572, -2.2603) (32.5572, -2.3417) knots 0 0 0 1 1 1
  spline S191 degree 2 poles (32.5572, -2.3417) (32.5572, -2.4638) (33.0863, -2.4638) knots 0 0 0 1 1 1
  spline S192 degree 2 poles (33.0863, -2.4638) (33.6651, -2.4638) (33.6651, -2.3439) knots 0 0 0 1 1 1
  spline S193 degree 2 poles (33.6651, -2.3439) (33.6651, -2.2264) (33.4186, -2.2264) knots 0 0 0 1 1 1
  line L347 (33.4186, -2.2264) -> (33.3146, -2.2286)
  line L348 (33.3146, -2.2286) -> (33.2377, -2.2309)
  line L349 (33.2377, -2.2309) -> (33.1857, -2.2309)
  line L350 (33.1857, -2.2309) -> (33.1857, -1.937)
  line L351 (31.9784, -0.8698) -> (32.5889, -0.8698)
  line L352 (32.5889, -0.8698) -> (33.6063, -1.469)
  line L353 (33.6063, -1.469) -> (33.6063, -1.1298)
  line L354 (33.6063, -1.1298) -> (33.3191, -1.1298)
  line L355 (33.3191, -1.1298) -> (33.3191, -0.8698)
  line L356 (33.3191, -0.8698) -> (34.2484, -0.8698)
  line L357 (34.2484, -0.8698) -> (34.2484, -1.8149)
  line L358 (34.2484, -1.8149) -> (33.5746, -1.8149)
  line L359 (33.5746, -1.8149) -> (32.5889, -1.1931)
  line L360 (32.5889, -1.1931) -> (32.5889, -1.521)
  line L361 (32.5889, -1.521) -> (32.8556, -1.521)
  line L362 (32.8556, -1.521) -> (32.8556, -1.781)
  line L363 (32.8556, -1.781) -> (31.9784, -1.781)
  line L364 (31.9784, -1.781) -> (31.9784, -0.8698)
  line L365 (31.9784, 0.3353) -> (32.5889, 0.3353)
  line L366 (32.5889, 0.3353) -> (32.5889, 0.2267)
  line L367 (32.5889, 0.2267) -> (34.3411, -0.022)
  spline S194 degree 2 poles (34.3411, -0.022) (35.0668, -0.126) (35.0668, -0.4448) knots 0 0 0 1 1 1
  spline S195 degree 2 poles (35.0668, -0.4448) (35.0668, -0.7703) (34.6147, -0.7703) knots 0 0 0 1 1 1
  spline S196 degree 2 poles (34.6147, -0.7703) (34.4632, -0.7703) (34.2959, -0.7455) knots 0 0 0 1 1 1
  line L368 (34.2959, -0.7455) -> (34.2959, -0.5329)
  spline S197 degree 2 poles (34.2959, -0.5329) (34.3592, -0.542) (34.4044, -0.542) knots 0 0 0 1 1 1
  spline S198 degree 2 poles (34.4044, -0.542) (34.54, -0.542) (34.54, -0.4493) knots 0 0 0 1 1 1
  spline S199 degree 2 poles (34.54, -0.4493) (34.54, -0.3634) (34.2959, -0.3181) knots 0 0 0 1 1 1
  line L369 (34.2959, -0.3181) -> (32.5889, -0.6528)
  line L370 (32.5889, -0.6528) -> (32.5889, -0.7681)
  line L371 (32.5889, -0.7681) -> (31.9784, -0.7681)
  line L372 (31.9784, -0.7681) -> (31.9784, -0.2277)
  line L373 (31.9784, -0.2277) -> (32.5889, -0.2277)
  line L374 (32.5889, -0.2277) -> (32.5889, -0.3407)
  line L375 (32.5889, -0.3407) -> (33.5769, -0.144)
  line L376 (33.5769, -0.144) -> (32.5889, -0.022)
  line L377 (32.5889, -0.022) -> (32.5889, -0.144)
  line L378 (32.5889, -0.144) -> (31.9784, -0.144)
  line L379 (31.9784, -0.144) -> (31.9784, 0.3353)
  line L380 (35.0176, 14.7406) -> (31.9676, 14.7406)
  line L381 (31.9676, 14.7406) -> (31.9676, 16.0936)
  spline S200 degree 2 poles (31.9676, 16.0936) (31.9676, 16.5004) (32.1326, 16.9258) (32.5487, 17.1792) (32.7998, 17.1792) knots 0 0 0 1 2 3 3 3
  spline S201 degree 2 poles (32.7998, 17.1792) (33.1253, 17.1792) (33.5693, 16.7585) (33.6297, 16.3214) knots 0 0 0 1 2 2 2
  spline S202 degree 2 poles (33.6297, 16.3214) (33.7064, 16.4795) (33.7808, 16.5632) knots 0 0 0 1 1 1
  spline S203 degree 2 poles (33.7808, 16.5632) (33.9436, 16.7399) (34.1877, 16.8979) knots 0 0 0 1 1 1
  line L382 (34.1877, 16.8979) -> (35.0176, 17.4257)
  line L383 (35.0176, 17.4257) -> (35.0176, 16.9212)
  line L384 (35.0176, 16.9212) -> (34.3829, 16.5167)
  spline S204 degree 2 poles (34.3829, 16.5167) (34.1086, 16.34) (33.818, 16.1122) (33.6995, 15.9309) (33.6762, 15.8379) knots 0 0 0 1 2 3 3 3
  spline S205 degree 2 poles (33.6762, 15.8379) (33.6623, 15.7681) (33.6623, 15.6124) knots 0 0 0 1 1 1
  line L385 (33.6623, 15.6124) -> (33.6623, 15.1451)
  line L386 (33.6623, 15.1451) -> (35.0176, 15.1451)
  line L387 (35.0176, 15.1451) -> (35.0176, 14.7406)
  line L388 (33.3136, 15.1451) -> (33.3136, 16.0122)
  spline S206 degree 2 poles (33.3136, 16.0122) (33.3136, 16.2889) (33.1997, 16.6004) (32.9463, 16.7631) (32.7998, 16.7631) knots 0 0 0 1 2 3 3 3
  spline S207 degree 2 poles (32.7998, 16.7631) (32.5836, 16.7631) (32.3047, 16.4493) (32.3047, 16.1099) knots 0 0 0 1 2 2 2
  line L389 (32.3047, 16.1099) -> (32.3047, 15.1451)
  line L390 (32.3047, 15.1451) -> (33.3136, 15.1451)
  line L391 (35.0176, 17.5675) -> (34.713, 17.5675)
  line L392 (34.713, 17.5675) -> (33.0997, 18.9716)
  spline S208 degree 2 poles (33.0997, 18.9716) (33.1113, 18.7321) (33.1113, 18.5485) knots 0 0 0 1 1 1
  line L393 (33.1113, 18.5485) -> (33.1113, 17.6511)
  line L394 (33.1113, 17.6511) -> (32.8068, 17.6511)
  line L395 (32.8068, 17.6511) -> (32.8068, 19.4551)
  line L396 (32.8068, 19.4551) -> (33.0555, 19.4551)
  line L397 (33.0555, 19.4551) -> (34.4573, 18.2579)
  line L398 (34.4573, 18.2579) -> (34.713, 18.0301)
  spline S209 degree 2 poles (34.713, 18.0301) (34.6944, 18.2811) (34.6944, 18.502) knots 0 0 0 1 1 1
  line L399 (34.6944, 18.502) -> (34.6944, 19.5225)
  line L400 (34.6944, 19.5225) -> (35.0176, 19.5225)
  line L401 (35.0176, 19.5225) -> (35.0176, 17.5675)
  line L402 (34.3039, 21.4079) -> (34.3527, 21.7961)
  spline S210 degree 2 poles (34.3527, 21.7961) (34.6921, 21.7031) (35.0664, 21.2079) (35.0664, 20.8244) knots 0 0 0 1 2 2 2
  spline S211 degree 2 poles (35.0664, 20.8244) (35.0664, 20.3385) (34.4689, 19.7713) (33.9319, 19.7713) knots 0 0 0 1 2 2 2
  spline S212 degree 2 poles (33.9319, 19.7713) (33.374, 19.7713) (32.758, 20.3455) (32.758, 20.8034) knots 0 0 0 1 2 2 2
  spline S213 degree 2 poles (32.758, 20.8034) (32.758, 21.2451) (33.3624, 21.8077) (33.9087, 21.8077) knots 0 0 0 1 2 2 2
  spline S214 degree 2 poles (33.9087, 21.8077) (33.9412, 21.8077) (34.0087, 21.8054) knots 0 0 0 1 1 1
  line L403 (34.0087, 21.8054) -> (34.0087, 20.1572)
  spline S215 degree 2 poles (34.0087, 20.1572) (34.3736, 20.1781) (34.7595, 20.5477) (34.7595, 20.8244) knots 0 0 0 1 2 2 2
  spline S216 degree 2 poles (34.7595, 20.8244) (34.7595, 21.0313) (34.541, 21.3218) (34.3039, 21.4079) knots 0 0 0 1 2 2 2
  line L404 (33.7018, 20.1781) -> (33.7018, 21.4125)
  spline S217 degree 2 poles (33.7018, 21.4125) (33.4228, 21.3869) (33.281, 21.2707) knots 0 0 0 1 1 1
  spline S218 degree 2 poles (33.281, 21.2707) (33.0648, 21.0917) (33.0648, 20.8058) knots 0 0 0 1 1 1
  spline S219 degree 2 poles (33.0648, 20.8058) (33.0648, 20.5477) (33.4112, 20.1967) (33.7018, 20.1781) knots 0 0 0 1 2 2 2
  line L405 (34.2086, 23.7093) -> (34.2574, 24.0766)
  spline S220 degree 2 poles (34.2574, 24.0766) (34.6363, 24.0162) (35.0664, 23.5187) (35.0664, 23.156) knots 0 0 0 1 2 2 2
  spline S221 degree 2 poles (35.0664, 23.156) (35.0664, 22.7027) (34.4736, 22.1518) (33.9203, 22.1518) knots 0 0 0 1 2 2 2
  spline S222 degree 2 poles (33.9203, 22.1518) (33.5623, 22.1518) (33.0253, 22.3889) (32.758, 22.8747) (32.758, 23.1583) knots 0 0 0 1 2 3 3 3
  spline S223 degree 2 poles (32.758, 23.1583) (32.758, 23.5187) (33.1229, 23.9766) (33.4577, 24.0417) knots 0 0 0 1 2 2 2
  line L406 (33.4577, 24.0417) -> (33.5135, 23.6768)
  spline S224 degree 2 poles (33.5135, 23.6768) (33.2903, 23.6256) (33.0648, 23.3606) (33.0648, 23.1746) knots 0 0 0 1 2 2 2
  spline S225 degree 2 poles (33.0648, 23.1746) (33.0648, 22.891) (33.4716, 22.5377) (33.911, 22.5377) knots 0 0 0 1 2 2 2
  spline S226 degree 2 poles (33.911, 22.5377) (34.355, 22.5377) (34.7595, 22.8794) (34.7595, 23.1537) knots 0 0 0 1 2 2 2
  spline S227 degree 2 poles (34.7595, 23.1537) (34.7595, 23.3745) (34.4899, 23.6698) (34.2086, 23.7093) knots 0 0 0 1 2 2 2
  line L407 (35.0176, 24.1998) -> (34.713, 24.1998)
  line L408 (34.713, 24.1998) -> (33.0997, 25.6039)